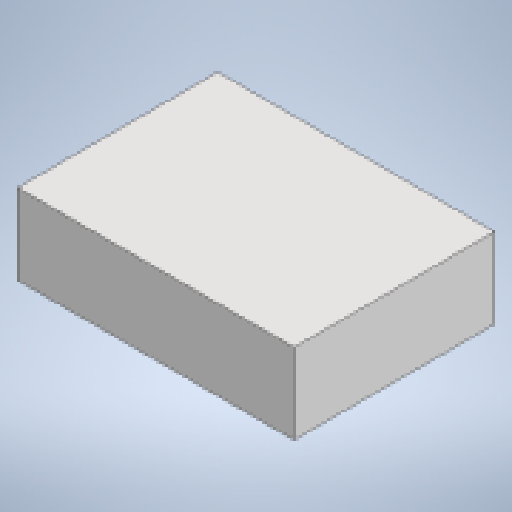
# Autodesk Inventor part: стена2
Saved by Autodesk Inventor 2023.1 (Build 271208000, 208)
## iProperties
Created: 2025-12-23
Part Number: стена2
Material: Типовые
Document SubType Name: Modeling
Designer: DELL
Density: 1 g/cm^3
Appearance: По умолчанию
Author: DELL
Autodesk Inventor part; units mm, degrees
ref_plane "YZ Plane" through (0, 0, 0) normal (1, 0, 0) x (0, 1, 0)
ref_plane "XZ Plane" through (0, 0, 0) normal (0, 1, 0) x (-1, 0, 0)
ref_plane "XY Plane" through (0, 0, 0) normal (0, 0, 1) x (1, 0, 0)
sketch "Эскиз1" plane through (0, 0, 0) normal (0, 0, 1) x (1, 0, 0)
  line L0 (27.6155, -8) -> (-27.6155, -8)
  line L1 (-27.6155, -8) -> (-27.6155, 8)
  line L2 (-27.6155, 8) -> (27.6155, 8)
  line L3 (27.6155, 8) -> (27.6155, -8)
  line L4 (27.6155, -8) -> (-27.6155, 8) construction
  line L5 (-27.6155, -8) -> (27.6155, 8) construction
  point P0 (0, 0)
  dimension "d0" = 55.231
  dimension "d1" = 16
  constraints: 12 end point, 2 midpoint, 2 parallel, 1 horizontal, 1 perpendicular
  measures "d0" distance of L1.end L2.end
  measures "d1" distance of L0.end L1.end
extrude "Выдавливание1" add sketch "Эскиз1" along normal blind 40
